nixal_reprap4040_inductiveMount (Autodesk Fusion 360 design; units mm, degrees)
Autodesk Fusion 360 part; units mm, degrees
sketch "Sketch1" plane through (0, 0, 0) normal (0, 1, 0) x (1, 0, 0)
  circle A0 centre (0, 0) radius 6.2
  circle A1 centre (0, 0) radius 11
  line L0 (-1.1288, 10.9419) -> (-48.1288, 10.9419)
  line L1 (-48.1288, 10.9419) -> (-48.1288, 6.9419)
  line L2 (-48.1288, 6.9419) -> (-1.1288, 6.9419)
  line L3 (-1.1288, 6.9419) -> (-1.1288, 10.9419)
  line L4 (-10.7088, 6.9419) -> (-10.7088, 10.9419)
  line L5 (-10.9899, 0.4722) -> (-10.7119, 6.9419)
  line L6 (-10.9899, -0.053) -> (-17.9945, 6.9419)
  dimension "d1" = 12.4
  dimension "d2" = 22
  dimension "d3" = 47
  dimension "d4" = 4
  constraint coincident A0.centre A1.centre
  constraint horizontal L0
  constraint vertical L1
  constraint horizontal L2
  constraint vertical L3
  constraint coincident A1
  constraint coincident L2 A0.centre
  constraint coincident L0
  constraint perpendicular L0 L4
  constraint coincident A1 A0.centre
  constraint tangent A1 L5
  measures "d1" diameter of A0
  measures "d2" diameter of A1
  measures "d4" distance of A0.centre
extrude "Extrude1" add sketch "Sketch1" along normal blind 8 contours A1 L0 L2 L4 | L0 L1 L2 L4
extrude "Extrude2" add sketch "Sketch1" along normal blind 8 contours A1 L2 L3 | A1 L2 L3 | A1 L2 L5 L6 | A1 L2 L5
extrude "Extrude3" add sketch "Sketch1" along normal blind -20 and the other way blind 0 contours L0 L1 L2 L4
sketch "Sketch2" plane through (0, 0, -6.9419) normal (0, 0, 1) x (1, 0, 0)
  line L0 (-10.7088, 0) -> (-17.9945, 0)
  line L1 (-17.9945, 8) -> (-48.1288, 8)
  line L2 (-48.1288, 8) -> (-48.1288, -20)
  line L3 (-48.1288, -20) -> (-10.7088, -20)
  line L4 (-10.7088, -20) -> (-10.7088, 0)
  circle A0 centre (-41.7088, -15) radius 1.6
  circle A1 centre (-16.7088, -15) radius 1.6
  line L5 (-17.9945, 0) -> (-17.9945, 8)
  dimension "d12" = 3.2
  dimension "d13" = 3.2
  dimension "d16" = 23
  dimension "d17" = 5
  dimension "d18" = 5
  dimension "d19" = 29.0087
  dimension "d20" = 25
  dimension "d21" = 6
  dimension "d22" = 7.3073
  measures "d12" diameter of A0
  measures "d13" diameter of A1
  measures "d16" distance of origin
  measures "d17" distance of L3
  measures "d18" distance of L3
  measures "d19" distance of origin
  measures "d22" distance of L2
extrude "Extrude4" cut sketch "Sketch2" against normal blind 10 contours A0 | A1
